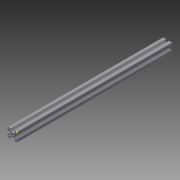
# Autodesk Inventor part: Balka
Saved by Autodesk Inventor 2015 (Build 190159000, 159)
## iProperties
Created: 2016-04-26
Part Number: Balka
Material: Generic
Document SubType Name: Modeling
Designer: Andreas
Density: 1 g/cm^3
Appearance: Default
Author: Andreas
Autodesk Inventor part; units mm, degrees
ref_plane "YZ Plane" through (0, 0, 0) normal (1, 0, 0) x (0, 1, 0)
ref_plane "XZ Plane" through (0, 0, 0) normal (0, 1, 0) x (-1, 0, 0)
ref_plane "XY Plane" through (0, 0, 0) normal (0, 0, 1) x (1, 0, 0)
sketch "Sketch1" plane through (0, 0, 0) normal (0, 1, 0) x (-1, 0, 0)
  line L0 (0, -1.5) -> (0, -9.8)
  line L1 (0, -9.8) -> (1.1, -9.8)
  line L2 (1.1, -9.8) -> (1.1, -10.9)
  line L3 (1.1, -10.9) -> (2.2, -10.9)
  line L4 (2.2, -10.9) -> (2.2, -6.75)
  line L5 (0, -28.5) -> (0, -20.2)
  line L6 (0, -20.2) -> (1.1, -20.2)
  line L7 (1.1, -20.2) -> (1.1, -19.1)
  line L8 (1.1, -19.1) -> (2.2, -19.1)
  line L9 (2.2, -19.1) -> (2.2, -23.25)
  line L10 (1.5, 0) -> (9.8, 0)
  line L11 (9.8, 0) -> (9.8, -1.1)
  line L12 (9.8, -1.1) -> (10.9, -1.1)
  line L13 (10.9, -1.1) -> (10.9, -2.2)
  line L14 (10.9, -2.2) -> (6.75, -2.2)
  line L15 (28.5, 0) -> (20.2, 0)
  line L16 (20.2, 0) -> (20.2, -1.1)
  line L17 (20.2, -1.1) -> (19.1, -1.1)
  line L18 (19.1, -1.1) -> (19.1, -2.2)
  line L19 (19.1, -2.2) -> (23.25, -2.2)
  line L20 (30, -1.5) -> (30, -9.8)
  line L21 (30, -9.8) -> (28.9, -9.8)
  line L22 (28.9, -9.8) -> (28.9, -10.9)
  line L23 (28.9, -10.9) -> (27.8, -10.9)
  line L24 (27.8, -10.9) -> (27.8, -6.75)
  line L25 (30, -28.5) -> (30, -20.2)
  line L26 (30, -20.2) -> (28.9, -20.2)
  line L27 (28.9, -20.2) -> (28.9, -19.1)
  line L28 (28.9, -19.1) -> (27.8, -19.1)
  line L29 (27.8, -19.1) -> (27.8, -23.25)
  line L30 (28.5, -30) -> (20.2, -30)
  line L31 (20.2, -30) -> (20.2, -28.9)
  line L32 (20.2, -28.9) -> (19.1, -28.9)
  line L33 (19.1, -28.9) -> (19.1, -27.8)
  line L34 (19.1, -27.8) -> (23.25, -27.8)
  line L35 (1.5, -30) -> (9.8, -30)
  line L36 (9.8, -30) -> (9.8, -28.9)
  line L37 (9.8, -28.9) -> (10.9, -28.9)
  line L38 (10.9, -28.9) -> (10.9, -27.8)
  line L39 (10.9, -27.8) -> (6.75, -27.8)
  line L40 (6.75, -2.2) -> (6.75, -6.75)
  line L41 (6.75, -6.75) -> (2.2, -6.75)
  line L42 (2.2, -23.25) -> (6.75, -23.25)
  line L43 (6.75, -23.25) -> (6.75, -27.8)
  line L44 (23.25, -27.8) -> (23.25, -23.25)
  line L45 (23.25, -23.25) -> (27.8, -23.25)
  line L46 (27.8, -6.75) -> (23.25, -6.75)
  line L47 (23.25, -2.2) -> (23.25, -6.75)
  line L48 (9.2, -9.2) -> (20.8, -9.2)
  line L49 (20.8, -9.2) -> (20.8, -20.8)
  line L50 (20.8, -20.8) -> (9.2, -20.8)
  line L51 (9.2, -20.8) -> (9.2, -9.2)
  line L52 (23.25, -6.75) -> (23.25, -5.194)
  line L53 (23.25, -6.75) -> (24.806, -6.75)
  line L54 (6.75, -6.75) -> (5.194, -6.75)
  line L55 (6.75, -6.75) -> (6.75, -5.194)
  line L56 (6.75, -23.25) -> (5.194, -23.25)
  line L57 (6.75, -23.25) -> (6.75, -24.806)
  line L58 (23.25, -23.25) -> (23.25, -24.806)
  line L59 (23.25, -23.25) -> (24.806, -23.25)
  line L60 (5.194, -23.25) -> (23.25, -5.194)
  line L61 (24.806, -6.75) -> (6.75, -24.806)
  circle A0 centre (15, -15) radius 3.4
  arc A1 (1.5, 0) -> (0, -1.5) centre (1.5, -1.5) ccw
  arc A2 (0, -28.5) -> (1.5, -30) centre (1.5, -28.5) ccw
  arc A3 (28.5, -30) -> (30, -28.5) centre (28.5, -28.5) ccw
  arc A4 (30, -1.5) -> (28.5, 0) centre (28.5, -1.5) ccw
  line L62 (27.5, -1.5) -> (25.85, -1.5)
  line L63 (24.85, -2.5) -> (24.85, -4.15)
  line L64 (25.85, -5.15) -> (27.5, -5.15)
  line L65 (28.5, -4.15) -> (28.5, -2.5)
  line L66 (27.5, -24.85) -> (25.85, -24.85)
  line L67 (24.85, -25.85) -> (24.85, -27.5)
  line L68 (25.85, -28.5) -> (27.5, -28.5)
  line L69 (28.5, -27.5) -> (28.5, -25.85)
  line L70 (4.15, -24.85) -> (2.5, -24.85)
  line L71 (1.5, -25.85) -> (1.5, -27.5)
  line L72 (2.5, -28.5) -> (4.15, -28.5)
  line L73 (5.15, -27.5) -> (5.15, -25.85)
  line L74 (4.15, -1.5) -> (2.5, -1.5)
  line L75 (1.5, -2.5) -> (1.5, -4.15)
  line L76 (2.5, -5.15) -> (4.15, -5.15)
  line L77 (5.15, -4.15) -> (5.15, -2.5)
  arc A5 (27.5, -5.15) -> (28.5, -4.15) centre (27.5, -4.15) ccw
  arc A6 (28.5, -2.5) -> (27.5, -1.5) centre (27.5, -2.5) ccw
  arc A7 (25.85, -1.5) -> (24.85, -2.5) centre (25.85, -2.5) ccw
  arc A8 (24.85, -4.15) -> (25.85, -5.15) centre (25.85, -4.15) ccw
  arc A9 (5.15, -2.5) -> (4.15, -1.5) centre (4.15, -2.5) ccw
  arc A10 (1.5, -4.15) -> (2.5, -5.15) centre (2.5, -4.15) ccw
  arc A11 (4.15, -5.15) -> (5.15, -4.15) centre (4.15, -4.15) ccw
  arc A12 (2.5, -1.5) -> (1.5, -2.5) centre (2.5, -2.5) ccw
  arc A13 (2.5, -24.85) -> (1.5, -25.85) centre (2.5, -25.85) ccw
  arc A14 (5.15, -25.85) -> (4.15, -24.85) centre (4.15, -25.85) ccw
  arc A15 (4.15, -28.5) -> (5.15, -27.5) centre (4.15, -27.5) ccw
  arc A16 (1.5, -27.5) -> (2.5, -28.5) centre (2.5, -27.5) ccw
  arc A17 (25.85, -24.85) -> (24.85, -25.85) centre (25.85, -25.85) ccw
  arc A18 (28.5, -25.85) -> (27.5, -24.85) centre (27.5, -25.85) ccw
  arc A19 (27.5, -28.5) -> (28.5, -27.5) centre (27.5, -27.5) ccw
  arc A20 (24.85, -27.5) -> (25.85, -28.5) centre (25.85, -27.5) ccw
  line L78 (24.806, -23.25) -> (6.75, -5.194)
  line L79 (23.25, -24.806) -> (5.194, -6.75)
  point P0 (0, 0)
  point P1 (0, -30)
  point P2 (9.2, -15)
  point P3 (0, -15)
  point P4 (15, 0)
  point P5 (15, -9.2)
  dimension "d52" = 9.8
  dimension "d61" = 6.8
  dimension "d62" = 1.5
  dimension "d75" = 1.5
  dimension "d76" = 1.5
  dimension "d81" = 1
  dimension "d82" = 1.556
  dimension "d83" = 1.556
  dimension "d84" = 1.556
  dimension "d85" = 1.556
  dimension "d86" = 1.556
  dimension "d87" = 1.556
  dimension "d88" = 1.556
  constraints: 160 end point, 40 point on circle, 40 tangent, 38 perpendicular, 21 centre point, 18 equal radius, 16 point on line, 15 parallel, 6 horizontal, 3 equal length, 2 horizontal alignment, 2 midpoint, 2 vertical, 2 vertical alignment
  measures "d52" distance of point (0, -30) L5.end
  measures "d61" diameter of A0
  measures "d62" radius of A1
  measures "d75" distance between parallel lines of L35 L72
  measures "d76" distance between parallel lines of L5 L71
  measures "d81" radius of A5
  measures "d82" distance of L44.end L58.end
  measures "d83" distance of L44.end L59.end
  measures "d84" distance of L40.end L54.end
  measures "d85" distance of L42.end L56.end
  measures "d86" distance of L42.end L57.end
  measures "d87" distance of L53.end L46.end
  measures "d88" distance of L46.end L52.end
extrude "Extrusion1" add sketch "Sketch1" along normal blind 500 contours A1 L10 L11 L12 L13 L14 L40 L41 L4 L3 L2 L1 L0 | L41 L40 L78 L48 L51 L79 | L79 A0 L60 L51 | L51 L48 L78 A0 L79 | L60 A0 L61 L50 L51 | L51 L50 L61 L43 L42 L60 | A0 L78 L60 L79 | L48 L60 A0 L78 | L42 L43 L39 L38 L37 L36 L35 A2 L5 L6 L7 L8 L9 | L60 L79 L61 A0 | L60 L78 L61 L79 | L60 L47 L46 L61 L49 L48 | L48 L49 L61 A0 L60 | L61 A0 L79 L50 | A0 L61 L78 L60 | L61 L78 A0 L79 | L47 L19 L18 L17 L16 L15 A4 L20 L21 L22 L23 L24 L46 | L79 A0 L78 L49 L50 | L50 L49 L78 L45 L44 L79 | L61 L49 L78 A0 | L44 L45 L29 L28 L27 L26 L25 A3 L30 L31 L32 L33 L34
sketch "Sketch2" plane through (0, 0, 0) normal (0, -1, 0) x (1, 0, 0)
  circle A0 centre (-15, -15) radius 3.5
  line L0 (-20.2, -30) -> (-9.8, -30)
  line L1 (-1.5, -30) -> (-9.8, -30) projected
  line L2 (-30, -9.8) -> (-30, -20.2)
  point P0 (0, 0)
  point P1 (-30, -15)
  point P2 (-15, -30)
  dimension "d91" = 7
  constraints: 4 end point, 2 midpoint, 1 centre point, 1 collinear, 1 horizontal alignment, 1 vertical, 1 vertical alignment
  measures "d91" diameter of A0
extrude "Extrusion2" cut sketch "Sketch2" against normal blind 500
sketch "Sketch3" plane through (0, 0, 0) normal (0, -1, 0) x (1, 0, 0)
  point P0 (0, 0)
sketch "Sketch4" plane through (-19.244, 0, -9.2) normal (0, 0, 1) x (1, 0, 0)
  point P0 (34.244, 485)
sketch "Sketch5" plane through (-19.244, 0, -9.2) normal (0, 0, 1) x (1, 0, 0)
  point P0 (-25.756, 15)
body "Solid1"
